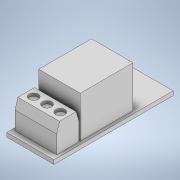
# Autodesk Inventor part: Relay w Breakout Board
Saved by Autodesk Inventor 2020.2 (Build 242310000, 310)
## iProperties
Created: 2020-04-13
Part Number: Relay w Breakout Board
Material: Generic
Document SubType Name: Modeling
Designer: Josiah
Density: 1 g/cm^3
Appearance: Default
Author: Josiah
Autodesk Inventor part; units mm, degrees
ref_plane "YZ Plane" through (0, 0, 0) normal (1, 0, 0) x (0, 1, 0)
ref_plane "XZ Plane" through (0, 0, 0) normal (0, 1, 0) x (-1, 0, 0)
ref_plane "XY Plane" through (0, 0, 0) normal (0, 0, 1) x (1, 0, 0)
sketch "Sketch1" plane through (0, 0, 0) normal (0, 1, 0) x (-1, 0, 0)
  line L0 (8.5, 21.5) -> (-8.5, 21.5)
  line L1 (-8.5, 21.5) -> (-8.5, -21.5)
  line L2 (-8.5, -21.5) -> (8.5, -21.5)
  line L3 (8.5, -21.5) -> (8.5, 21.5)
  line L4 (-8.5, 21.5) -> (8.5, -21.5) construction
  point P0 (0, 0)
  point P1 (0, 0)
  dimension "d0" = 43
  dimension "d1" = 17
  constraints: 10 end point, 2 parallel, 1 coincident, 1 horizontal, 1 midpoint, 1 perpendicular
  measures "d0" distance of L2.end L0.start
  measures "d1" distance of L1.end L2.end
extrude "Extrusion1" add sketch "Sketch1" along normal blind 1.5
sketch "Sketch2" plane through (0, 1.5, 0) normal (0, 1, 0) x (1, 0, 0)
  line L0 (-7.5, -11) -> (7.5, -11)
  line L1 (7.5, -11) -> (7.5, 8)
  line L2 (7.5, 8) -> (-7.5, 8)
  line L3 (-7.5, 8) -> (-7.5, -11)
  line L4 (-8.5, -21.5) -> (8.5, -21.5) projected
  point P0 (0, 0)
  dimension "d4" = 19
  dimension "d5" = 15
  dimension "d6" = 7.5
  dimension "d8" = 10.5
  constraints: 8 end point, 2 parallel, 1 horizontal, 1 perpendicular
  measures "d4" distance of L2.end L0.start
  measures "d5" distance of L1.end L2.end
  measures "d6" distance from line of point (0, 0) L3
  measures "d8" distance between parallel lines of L0 L4
extrude "Extrusion2" add sketch "Sketch2" along normal blind 15
sketch "Sketch3" plane through (0, 1.5, 0) normal (0, 1, 0) x (1, 0, 0)
  line L0 (7.5, -11.5) -> (-7.5, -11.5)
  line L1 (-7.5, -11.5) -> (-7.5, -19.5)
  line L2 (-7.5, -19.5) -> (7.5, -19.5)
  line L3 (7.5, -19.5) -> (7.5, -11.5)
  line L4 (-7.5, -11) -> (7.5, -11) projected
  point P0 (0, 0)
  dimension "d11" = 15
  dimension "d12" = 8
  dimension "d13" = 0.5
  dimension "d14" = 7.5
  constraints: 8 end point, 2 parallel, 1 horizontal, 1 perpendicular
  measures "d11" distance of L1.end L2.end
  measures "d12" distance of L2.end L0.start
  measures "d13" distance between parallel lines of L0 L4
  measures "d14" distance from line of point (0, 0) L1
extrude "Extrusion3" add sketch "Sketch3" along normal blind 10
chamfer "Chamfer1" distance 1 distance2 3.5 1 edges at (0, 11.5, 19.5) measured on face at (2.5, 11.5, 16.8333)
chamfer "Chamfer2" distance 1 distance2 3.5 1 edges at (0, 11.5, 11.5) measured on face at (2.5, 11.5, 16.1667)
sketch "Sketch4" plane through (0, 11.5, 0) normal (0, 1, 0) x (1, 0, 0)
  circle A0 centre (-4.8, -15.5) radius 1.65
  line L0 (-7.5, -12.5) -> (-7.5, -18.5) projected
  line L1 (-3.2324, -14.8041) -> (3.2927, -14.8041) construction
  circle A1 centre (0, -15.5) radius 1.65
  circle A2 centre (4.8, -15.5) radius 1.65
  point P0 (0, 0)
  dimension "d23" = 3.3
  dimension "d24" = 2.7
  dimension "d27" = 4.8
  dimension "d32" = 6
  dimension "d33" = 3
  constraints: 3 centre point, 2 end point, 2 horizontal, 4 other
  measures "d23" diameter of A0
  measures "d24" distance from line of A0.centre L0
  measures "d27" distance of A0.centre A1.centre
  measures "d32" distance of L0.start L0.end
  measures "d33" vertical distance of L0.start A0.centre
extrude "Extrusion4" cut sketch "Sketch4" against normal blind 1
equation "\"d6\" = 0.5 * d5"
equation "\"d14\" = 0.5 * d11"
equation "\"d33\" = 0.5 * d32"
body "Solid1"
